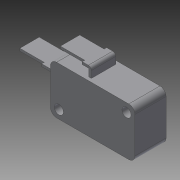
# Autodesk Inventor part: LimitSwitch
Saved by Autodesk Inventor 2014 SP1 (Build 180222100, 222)
## iProperties
Created: 2013-03-19
Part Number: LimitSwitch
Material: Generic
Document SubType Name: Modeling
Designer: ThatOtherGuy
Density: 1 g/cm^3
Appearance: Default
Author: ThatOtherGuy
Autodesk Inventor part; units mm, degrees
ref_plane "YZ Plane" through (0, 0, 0) normal (1, 0, 0) x (0, 1, 0)
ref_plane "XZ Plane" through (0, 0, 0) normal (0, 1, 0) x (-1, 0, 0)
ref_plane "XY Plane" through (0, 0, 0) normal (0, 0, 1) x (1, 0, 0)
sketch "Sketch1" plane through (0, 0, 0) normal (0, 1, 0) x (-1, 0, 0)
  circle A0 centre (2.75, 13.05) radius 1.5
  circle A1 centre (24.95, 2.75) radius 1.5
  line L0 (2, 15.8) -> (25.7, 15.8)
  line L1 (27.7, 13.8) -> (27.7, 2)
  line L2 (25.7, 0) -> (2, 0)
  line L3 (0, 2) -> (0, 13.8)
  arc A2 (0, 2) -> (2, 0) centre (2, 2) ccw
  arc A3 (25.7, 0) -> (27.7, 2) centre (25.7, 2) ccw
  arc A4 (27.7, 13.8) -> (25.7, 15.8) centre (25.7, 13.8) ccw
  arc A5 (2, 15.8) -> (0, 13.8) centre (2, 13.8) ccw
  point P0 (0, 0)
  point P1 (0, 0)
  point P2 (0, 0)
  dimension "d0" = 10.3
  dimension "d1" = 22.2
  dimension "d2" = 2.75
  dimension "d3" = 2.75
  dimension "d4" = 2.75
  dimension "d5" = 2.75
  dimension "d6" = 3
  dimension "d7" = 2
  constraints: 8 end point, 8 point on circle, 8 tangent, 6 centre point, 4 equal radius, 2 parallel, 2 point on line, 1 coincident, 1 horizontal, 1 perpendicular
  measures "d0" vertical distance of A1.centre A0.centre
  measures "d1" horizontal distance of A1.centre A0.centre
  measures "d2" distance from line of L2 A1.centre
  measures "d3" distance from line of A1.centre L1
  measures "d4" distance from line of L0 A0.centre
  measures "d5" distance from line of L3 A0.centre
  measures "d6" diameter of A1
  measures "d7" radius of A2
extrude "Extrusion1" add sketch "Sketch1" along normal blind 10.25
sketch "Sketch2" plane through (-2, 0, 0) normal (0, 0, -1) x (-1, 0, 0)
  line L0 (0, 0) -> (23.7, 0) projected
  line L1 (0, 10.25) -> (23.7, 10.25) projected
  line L2 (0, 0) -> (0, 10.25) projected
  line L3 (3.5, 7.25) -> (6.25, 7.25)
  line L4 (6.25, 7.25) -> (6.25, 3)
  line L5 (6.25, 3) -> (3.5, 3)
  line L6 (3.5, 3) -> (3.5, 7.25)
  point P0 (-2, 0)
  dimension "d10" = 4.25
  dimension "d12" = 2.75
  dimension "d13" = 3
  dimension "d14" = 3
  dimension "d15" = 3.5
  constraints: 8 end point, 2 parallel, 1 horizontal, 1 perpendicular
  measures "d10" distance of L3.end L4.end
  measures "d12" distance of L4.end L5.end
  measures "d13" distance between parallel lines of L1 L3
  measures "d14" distance between parallel lines of L0 L5
  measures "d15" distance between parallel lines of L2 L6
extrude "Extrusion2" add sketch "Sketch2" along normal blind 2.5
sketch "Sketch3" plane through (-27.7, 0, 2) normal (-1, 0, 0) x (0, 0, 1)
  line L0 (0, 0) -> (11.8, 0) projected
  line L1 (0, 10.25) -> (11.8, 10.25) projected
  line L2 (9, 9.125) -> (9.8, 9.125)
  line L3 (9.8, 9.125) -> (9.8, 1.125)
  line L4 (9.8, 1.125) -> (9, 1.125)
  line L5 (9, 1.125) -> (9, 9.125)
  line L6 (-2, 0) -> (-2, 10.25) projected
  dimension "d18" = 8
  dimension "d20" = 0.8
  dimension "d21" = 1.125
  dimension "d22" = 1.125
  dimension "d23" = 11
  constraints: 8 end point, 2 parallel, 1 horizontal, 1 perpendicular
  measures "d18" distance of L2.end L3.end
  measures "d20" distance of L2.start L2.end
  measures "d21" distance between parallel lines of L1 L2
  measures "d22" distance between parallel lines of L0 L4
  measures "d23" distance between parallel lines of L6 L5
extrude "Extrusion3" add sketch "Sketch3" along normal blind 12
sketch "Sketch5" plane through (-25.7, 0, 15.8) normal (0, 0, 1) x (1, 0, 0)
  line L0 (0, 0) -> (23.7, 0) projected
  line L1 (23.7, 0) -> (23.7, 10.25) projected
  line L2 (0, 10.25) -> (23.7, 10.25) projected
  line L3 (9.5, 9.125) -> (10.3, 9.125)
  line L4 (10.3, 9.125) -> (10.3, 1.125)
  line L5 (10.3, 1.125) -> (9.5, 1.125)
  line L6 (9.5, 1.125) -> (9.5, 9.125)
  line L7 (0, 0) -> (0, 10.25) projected
  point P0 (25.7, 0)
  dimension "d29" = 8
  dimension "d31" = 0.8
  dimension "d33" = 1.125
  dimension "d34" = 1.125
  dimension "d49" = 9.5
  dimension "d50" = 13.4
  constraints: 8 end point, 2 parallel, 1 horizontal, 1 perpendicular
  measures "d29" distance of L3.end L4.end
  measures "d31" distance of L3.start L3.end
  measures "d33" distance between parallel lines of L2 L3
  measures "d34" distance between parallel lines of L0 L5
  measures "d49" distance between parallel lines of L7 L6
  measures "d50" distance between parallel lines of L1 L4
extrude "Extrusion5" add sketch "Sketch5" along normal blind 3.25 contours L3 L4 L5 L6
sketch "Sketch6" plane through (-15.4, 1.125, 15.8) normal (1, 0, 0) x (0, 0, -1)
  line L0 (0, 0) -> (-3.25, 0) projected
  line L1 (-3.25, 8) -> (-2.45, 8)
  line L2 (-2.45, 8) -> (-2.45, 0)
  line L3 (-2.45, 0) -> (-3.25, 0)
  line L4 (-3.25, 0) -> (-3.25, 8)
  point P0 (15.8, -1.125)
  dimension "d37" = 0.8
  constraints: 8 end point, 2 parallel, 1 horizontal, 1 perpendicular, 1 point on line
  measures "d37" distance between parallel lines of L4 L2
extrude "Extrusion6" add sketch "Sketch6" against normal blind 11
fillet "Fillet1" radius 1 1 edges at (-15.4, 5.125, 19.05)
fillet "Fillet2" radius 0.25 1 edges at (-16.2, 5.125, 18.25)
sketch "Sketch9" plane through (-25.7, 0, 19.05) normal (0, 0, 1) x (1, 0, 0)
  line L0 (9.3, 9.125) -> (-0.7, 9.125) projected
  line L1 (-0.7, 1.125) -> (-0.7, 9.125) projected
  line L2 (9.3, 1.125) -> (-0.7, 1.125) projected
  line L3 (7.3, 9.125) -> (7.3, 8.3)
  line L4 (7.3, 8.3) -> (-0.7, 8.3)
  line L5 (7.3, 1.125) -> (7.3, 1.95)
  line L6 (7.3, 1.95) -> (-0.7, 1.95)
  line L7 (10.3, 1.125) -> (10.3, 9.125) projected
  point P0 (25.7, 0)
  dimension "d51" = 6.35
  dimension "d53" = 3
  constraints: 8 end point, 5 perpendicular, 4 point on line, 2 equal length
  measures "d51" distance between parallel lines of L4 L6
  measures "d53" distance between parallel lines of L7 L3
extrude "Extrusion9" cut sketch "Sketch9" against normal up to next
sketch "Sketch10" plane through (-27.7, 1.125, 11.8) normal (0, 0, 1) x (1, 0, 0)
  line L0 (0, 8) -> (-12, 8) projected
  line L1 (-12, 0) -> (-12, 8) projected
  line L2 (0, 0) -> (-12, 0) projected
  line L3 (-12, 7.175) -> (-4, 7.175)
  line L4 (-4, 7.175) -> (-4, 8)
  line L5 (-4, 0) -> (-4, 0.825)
  line L6 (-4, 0.825) -> (-12, 0.825)
  point P0 (27.7, -1.125)
  dimension "d56" = 6.35
  dimension "d57" = 8
  constraints: 8 end point, 4 point on line, 2 equal length, 2 perpendicular, 1 collinear, 1 parallel
  measures "d56" distance between parallel lines of L3 L6
  measures "d57" distance of L3.start L3.end
extrude "Extrusion10" cut sketch "Sketch10" against normal up to next
equation "\"d3\" = d2"
equation "\"d4\" = d2"
equation "\"d5\" = d2"
equation "\"d13\" = d14"
equation "\"d21\" = d22"
equation "\"d33\" = d34"
body "Solid1"
